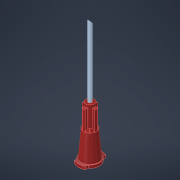
# Autodesk Inventor part: CH_01_0030_needle_1
Saved by Autodesk Inventor 2022 (Build 260153000, 153)
## iProperties
Created: 2022-03-16
Part Number: CH_01_0030_needle_1
Material: Generic
Document SubType Name: Modeling
Designer: Tomasz Krakowski
Density: 1 g/cm^3
Appearance: Default
Author: Tomasz Krakowski
Autodesk Inventor part; units mm, degrees
ref_plane "YZ Plane" through (0, 0, 0) normal (1, 0, 0) x (0, 1, 0)
ref_plane "XZ Plane" through (0, 0, 0) normal (0, 1, 0) x (-1, 0, 0)
ref_plane "XY Plane" through (0, 0, 0) normal (0, 0, 1) x (1, 0, 0)
sketch "Sketch1" plane through (0, 0, 0) normal (0, 1, 0) x (-1, 0, 0)
  circle A0 centre (0, 0) radius 0.525
  circle A1 centre (0, 0) radius 0.625
  dimension "d0" = 1.25
  dimension "d1" = 0.1
  constraints: 2 centre point, 2 coincident
  measures "d0" diameter of A1
  measures "d1" radial gap between concentric circles of A1 A0
extrude "Extrusion1" add sketch "Sketch1" along normal blind 25
sketch "Sketch2" plane through (0, 0, 0) normal (1, 0, 0) x (0, 1, 0)
  line L0 (25, -0.625) -> (25, 0.625) construction
  line L1 (25, 0.625) -> (23.5, -0.625)
  line L2 (25, 0.625) -> (25, -0.625)
  line L3 (25, -0.625) -> (23.5, -0.625)
  point P0 (0, 0)
  dimension "d4" = 1.5
  constraints: 6 end point, 1 collinear, 1 horizontal
  measures "d4" horizontal distance of L0.end L1.end
extrude "Extrusion2" cut sketch "Sketch2" along normal through all both and the other way through all
sketch "Sketch3" plane through (0, 0, 0) normal (0, -1, 0) x (1, 0, 0)
  circle A0 centre (0, 0) radius 1.5
  circle A1 centre (0, 0) radius 0.625
  circle A2 centre (0, 0) radius 0.625 construction
  dimension "d7" = 3
  constraints: 2 centre point, 2 coincident, 1 concentric
  measures "d7" diameter of A0
extrude "Extrusion3" add sketch "Sketch3" along normal blind 1 separate body
sketch "Sketch4" plane through (0, -1, 0) normal (0, -1, 0) x (1, 0, 0)
  line L0 (0.5, -1.4142) -> (0.5, -2.25)
  line L1 (0.5, -2.25) -> (-0.5, -2.25)
  line L2 (-0.5, -2.25) -> (-0.5, -1.4142)
  arc A0 (-0.5, -1.4142) -> (0.5, -1.4142) centre (0, 0) ccw
  circle A1 centre (0, 0) radius 1.5 projected
  line L3 (1.4142, 0.5) -> (2.25, 0.5)
  line L4 (2.25, 0.5) -> (2.25, -0.5)
  line L5 (2.25, -0.5) -> (1.4142, -0.5)
  arc A2 (1.4142, -0.5) -> (1.4142, 0.5) centre (0, 0) ccw
  line L6 (-0.5, 1.4142) -> (-0.5, 2.25)
  line L7 (-0.5, 2.25) -> (0.5, 2.25)
  line L8 (0.5, 2.25) -> (0.5, 1.4142)
  arc A3 (0.5, 1.4142) -> (-0.5, 1.4142) centre (0, 0) ccw
  line L9 (-1.4142, -0.5) -> (-2.25, -0.5)
  line L10 (-2.25, -0.5) -> (-2.25, 0.5)
  line L11 (-2.25, 0.5) -> (-1.4142, 0.5)
  arc A4 (-1.4142, 0.5) -> (-1.4142, -0.5) centre (0, 0) ccw
  circle A5 centre (0, 0) radius 1.5 construction
  circle A6 centre (0, 0) radius 1.5 construction
  circle A7 centre (0, 0) radius 1.5
  circle A8 centre (0, 0) radius 1.3
  dimension "d20" = 2.25
  dimension "d21" = 1
  dimension "d24" = 360
  dimension "d26" = 0.2
  constraints: 24 end point, 8 centre point, 8 point on circle, 5 coincident, 3 concentric, 2 vertical, 1 parallel, 1 perpendicular, 37 other
  measures "d20" distance from line of L1 point (0, 0)
  measures "d21" distance between parallel lines of L2 L0
  measures "d26" radial gap between concentric circles of A1 A8
extrude "Extrusion4" add sketch "Sketch4" along normal blind 7 bodies 2
sketch "Sketch5" plane through (0, 0, 0) normal (0, 0, 1) x (1, 0, 0)
  line L0 (1.3, -8) -> (-1.3, -8) construction
  line L1 (-1.3, -8) -> (-2.1, -18)
  line L2 (-2.1, -18) -> (-3.25, -18)
  line L3 (-3.25, -18) -> (-3.25, -17)
  line L4 (-3.25, -17) -> (-3, -17)
  line L5 (-2.25, -8) -> (-1.4142, -8) construction
  line L6 (-3, -17) -> (-2.25, -8)
  line L7 (-2.25, -8) -> (-1.3, -8)
  line L8 (0, -26.6) -> (0, 33.6) projected
  point P0 (0, 0)
  dimension "d27" = 2.1
  dimension "d28" = 3.25
  dimension "d29" = 3
  dimension "d30" = 9
  dimension "d31" = 1
  constraints: 12 end point, 2 horizontal, 2 perpendicular
  measures "d27" horizontal distance of L1.end point (0, 0)
  measures "d28" distance from line of point (0, 0) L3
  measures "d29" horizontal distance of point (0, 0) L4.end
  measures "d30" distance from line of L0 L3.end
  measures "d31" distance from line of L4.end L2
revolve "Revolution1" add sketch "Sketch5" angle 360 about axis through (0, -10, 0) along (0, 1, 0) bodies 2
chamfer "Chamfer1" distance 0.25 angle 45 4 edges at (2.25, -1, 0) (0, -1, -2.25) (-2.25, -1, 0) (0, -1, 2.25)
chamfer "Chamfer2" distance 0.75 angle 45 4 edges at (1.0607, -8, 1.0607) (1.0607, -8, -1.0607) (-1.0607, -8, -1.0607) (-1.0607, -8, 1.0607)
sketch "Sketch6" plane through (0, -18, 0) normal (0, -1, 0) x (1, 0, 0)
  circle A0 centre (0, 0) radius 3.25 construction
  line L0 (-1.875, -3.5333) -> (-2, -2.5617)
  circle A1 centre (0, 0) radius 3.25 construction
  line L1 (-3.25, 0) -> (0, 0) construction
  line L2 (0, -3.25) -> (0, 0) construction
  line L3 (1.875, -3.5333) -> (2, -2.5617)
  line L4 (-1.875, 3.5333) -> (-2, 2.5617)
  line L5 (1.875, 3.5333) -> (2, 2.5617)
  arc A2 (-1.875, -3.5333) -> (1.875, -3.5333) centre (0, 0) ccw
  arc A3 (1.875, 3.5333) -> (-1.875, 3.5333) centre (0, 0) ccw
  arc A4 (2, 2.5617) -> (-2, 2.5617) centre (0, 0) ccw
  arc A5 (-2, -2.5617) -> (2, -2.5617) centre (0, 0) ccw
  dimension "d40" = 1.875
  dimension "d41" = 2
  dimension "d42" = 4
  constraints: 12 end point, 10 point on circle, 6 symmetric about line, 4 centre point, 2 coincident, 1 concentric, 1 horizontal, 1 vertical
  measures "d40" horizontal distance of L0.start point (0, 0)
  measures "d41" horizontal distance of point (0, 0) L0.end
  measures "d42" radius of A2
extrude "Extrusion5" add sketch "Sketch6" against normal up to surface (1 mm away) bodies 2
body "Solid1"
body "Solid2"
